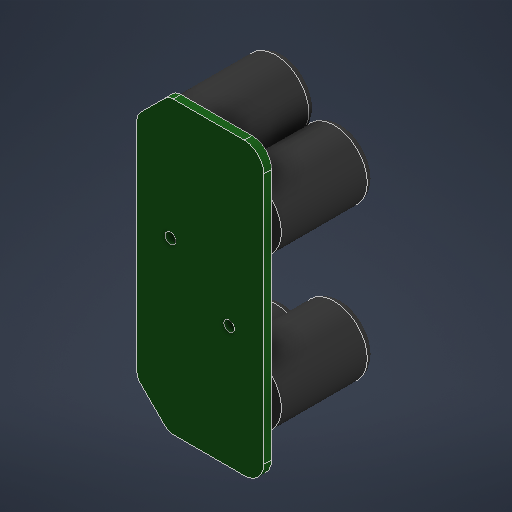
# Autodesk Inventor part: Solenoid Board
Saved by Autodesk Inventor 2026.1 (Build 301233020, 233B)
## iProperties
Created: 2025-11-08
Part Number: Solenoid Board
Material: Generic
Document SubType Name: Modeling
Designer: Bahaa
Density: 1 g/cm^3
Appearance: Default
Author: Bahaa
Autodesk Inventor part; units mm, degrees
ref_plane "YZ Plane" through (0, 0, 0) normal (1, 0, 0) x (0, 1, 0)
ref_plane "XZ Plane" through (0, 0, 0) normal (0, 1, 0) x (-1, 0, 0)
ref_plane "XY Plane" through (0, 0, 0) normal (0, 0, 1) x (1, 0, 0)
sketch "Sketch1" plane through (0, 0, 0) normal (0, 1, 0) x (-1, 0, 0)
  line L0 (16.25, 11) -> (-16.25, 11)
  line L1 (-16.25, 11) -> (-16.25, -11)
  line L2 (-16.25, -11) -> (16.25, -11)
  line L3 (16.25, -11) -> (16.25, 11)
  line L4 (16.25, 11) -> (-16.25, -11) construction
  line L5 (-16.25, 11) -> (16.25, -11) construction
  line L6 (16.25, 11) -> (7.65, 11)
  line L7 (7.65, 11) -> (7.65, 6) construction
  line L8 (7.65, 6) -> (16.25, 6) construction
  line L9 (16.25, 6) -> (16.25, 11)
  line L10 (-16.25, -11) -> (-7.35, -11)
  line L11 (-7.35, -11) -> (-7.35, -6) construction
  line L12 (-16.25, -6) -> (-16.25, -11)
  circle A0 centre (7.65, 6) radius 1.35
  circle A1 centre (-7.35, -6) radius 1.35
  line L13 (8.1983, 37.2) -> (16.25, 29.1483)
  line L14 (8.1983, 37.2) -> (-16.25, 37.2)
  line L15 (-16.25, 37.2) -> (-16.25, 11)
  line L16 (16.25, 0) -> (-16.25, 0) construction
  line L17 (16.25, -29.1483) -> (16.25, 7.9473)
  line L18 (8.1983, -37.2) -> (16.25, -29.1483)
  line L19 (8.1983, -37.2) -> (-16.25, -37.2)
  line L20 (-16.25, -37.2) -> (-16.25, -11)
  line L21 (16.25, 11) -> (16.25, 29.1483)
  circle A2 centre (4.75, 27.5942) radius 8.5
  circle A3 centre (-10.25, 19.5) radius 8.5
  circle A4 centre (4.75, -27.5942) radius 8.5
  circle A5 centre (-10.25, -19.5) radius 8.5
  point P0 (0, 0)
  point P1 (16.25, -11)
  point P2 (0, 0)
  dimension "d0" = 32.5
  dimension "d1" = 22
  dimension "d2" = 8.6
  dimension "d3" = 5
  dimension "d5" = 5
  dimension "d6" = 2.7
  dimension "d7" = 2.7
  dimension "d17" = 26.2
  dimension "d22" = 23.6
  dimension "d23" = 135
  dimension "d25" = 11.3869
  dimension "d27" = 135
  dimension "d30" = 56
  dimension "d31" = 17
  dimension "d32" = 21
  dimension "d33" = 17
  dimension "d34" = 39
  dimension "d35" = 6
  constraints: 44 end point, 6 centre point, 5 midpoint, 5 parallel, 5 symmetric about line, 4 horizontal, 3 perpendicular, 2 coincident, 2 collinear, 2 other
  measures "d0" distance of L2.end L1.end
  measures "d1" distance of L2.end L0.start
  measures "d2" distance of L8.end L7.end
  measures "d3" distance of L7.end L6.end
  measures "d5" distance of L11.end L10.end
  measures "d6" diameter of A0
  measures "d7" diameter of A1
  measures "d17" distance of L14.end L0.end
  measures "d22" distance from line of L3 L11.end
  measures "d23" angle of L13 L21
  measures "d25" distance of L13.start L13.end
  measures "d27" angle of L18 L17
  measures "d30" diameter of A2.centre point (0, 0)
  measures "d31" diameter of A2
  measures "d32" distance from line of L15 A2.centre
  measures "d33" diameter of A3
  measures "d34" diameter of A3.centre L16
  measures "d35" distance from line of L15 A3.centre
extrude "Extrusion1" add sketch "Sketch1" along normal blind 2 contours L3 L2 L1 L0 | L0 A3 L15 L14 L13 L21 | L0 L15 A3 | A3 L15 | L17 L18 L19 L20 A5 L2 | L2 A5 L20 | A5 L20 | A2 | A4 picked at (-10.5425, 20.2212) picked at (-11.2683, -17.9197)
fillet "Fillet1" radius 3 4 edges at (-8.1983, 1, 37.2) (-16.25, 1, 29.1483) (-16.25, 1, -29.1483) (-8.1983, 1, -37.2)
fillet "Fillet2" radius 5 2 edges at (16.25, 1, 37.2) (16.25, 1, -37.2)
extrude "Extrusion2" add sketch "Sketch1" along normal blind 24 from surface at 2 contours A3 L15 | A3 L15 | A5 L20 | L20 A5 | A2 | A4
fillet "Fillet3" radius 2 4 edges at (18.75, 26, 19.5) (3.75, 26, 27.5942) (18.75, 26, -19.5) (3.75, 26, -27.5942)
equation "\"d27\" = d23"
body "Solid1"
